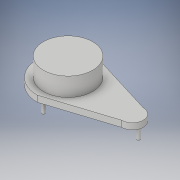
# Autodesk Inventor part: LIDAR-Sensor
Saved by Autodesk Inventor 2019.5 (Build 235369000, 369)
## iProperties
Created: 2021-10-01
Part Number: LIDAR-Sensor
Material: Generisch
Document SubType Name: Modeling
Designer: mritt
Density: 1 g/cm^3
Appearance: Vorgabe
Author: mritt
Autodesk Inventor part; units mm, degrees
ref_plane "YZ Plane" through (0, 0, 0) normal (1, 0, 0) x (0, 1, 0)
ref_plane "XZ Plane" through (0, 0, 0) normal (0, 1, 0) x (-1, 0, 0)
ref_plane "XY Plane" through (0, 0, 0) normal (0, 0, 1) x (1, 0, 0)
sketch "Skizze1" plane through (0, 0, 0) normal (0, 1, 0) x (-1, 0, 0)
  arc A0 (112.1495, -122.8972) -> (112.1495, -22.8972) centre (112.1495, -72.8972) ccw
  circle A1 centre (8.4112, -73.6215) radius 17.5
  line L0 (112.1495, -122.8972) -> (8.4112, -91.1215)
  line L1 (112.1495, -22.8972) -> (8.4112, -56.1215)
  point P0 (0, 0)
  dimension "d0" = 50
  dimension "d1" = 35
  constraints: 4 end point, 4 point on circle, 2 centre point
  measures "d0" radius of A0
  measures "d1" diameter of A1
extrude "Extrusion1" add sketch "Skizze1" along normal blind 10
sketch "Skizze2" plane through (0, 10, 0) normal (0, 1, 0) x (1, 0, 0)
  arc A0 (-112.1495, 122.8972) -> (-112.1495, 22.8972) centre (-112.1495, 72.8972) ccw projected
  circle A1 centre (-112.1495, 72.8972) radius 40
  point P0 (0, 0)
  dimension "d4" = 80
  constraints: 1 centre point, 1 coincident
  measures "d4" diameter of A1
extrude "Extrusion2" add sketch "Skizze2" along normal blind 30
sketch "Skizze3" plane through (0, 0, 0) normal (0, -1, 0) x (1, 0, 0)
  circle A0 centre (-112.1495, -112.8972) radius 2.5
  circle A1 centre (-112.1495, -32.8972) radius 2.5
  circle A2 centre (1.5888, -73.3753) radius 2.5
  arc A3 (-8.4112, -91.1215) -> (-8.4112, -56.1215) centre (-8.4112, -73.6215) ccw projected
  circle A4 centre (-112.1495, -72.8972) radius 40 projected
  point P0 (0, 0)
  dimension "d7" = 5
  dimension "d8" = 5
  dimension "d9" = 5
  dimension "d10" = 10
  dimension "d11" = 40
  dimension "d12" = 0
  dimension "d13" = 40
  constraints: 3 centre point, 1 vertical alignment, 1 other
  measures "d7" diameter of A0
  measures "d8" diameter of A1
  measures "d9" diameter of A2
  measures "d10" horizontal distance of A3.centre A2.centre
  measures "d11" distance of point (-112.15, -72.897) A0.centre
  measures "d12" horizontal distance of point (-112.15, -72.897) A0.centre
  measures "d13" distance of point (-112.15, -72.897) A1.centre
extrude "Extrusion3" add sketch "Skizze3" along normal blind 20 contours A0 A4 | A4 A0 | A4 A1 | A1 A4 | A2
